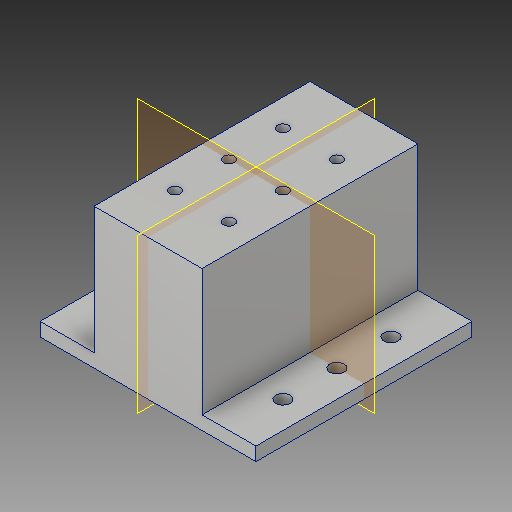
# Autodesk Inventor part: SupportPlateMotorMountV01
Saved by Autodesk Inventor 2017 (Build 210142000, 142)
## iProperties
Created: 2016-02-07
Part Number: SupportPlateMotorMountV01
Material: Aluminum 6061
Document SubType Name: Modeling
Designer: steele
Density: 2.7 g/cm^3
Appearance: Aluminum - Flat
Author: steele
Autodesk Inventor part; units mm, degrees
ref_plane "XZ Plane" through (0, 0, 0) normal (0, 1, 0) x (-1, 0, 0)
sketch "Sketch1" plane through (0, 0, 0) normal (0, 1, 0) x (-1, 0, 0)
  line L0 (50.8, 50.8) -> (-50.8, 50.8)
  line L1 (-50.8, 50.8) -> (-50.8, -50.8)
  line L2 (-50.8, -50.8) -> (50.8, -50.8)
  line L3 (50.8, -50.8) -> (50.8, 50.8)
  line L4 (50.8, 50.8) -> (-50.8, -50.8) construction
  line L5 (-50.8, 50.8) -> (50.8, -50.8) construction
  point P0 (0, 0)
  dimension "d0" = 101.6
  dimension "d1" = 101.6
  constraints: 12 end point, 2 midpoint, 2 parallel, 1 horizontal, 1 perpendicular
  measures "d0" distance of L2.end L0.start
  measures "d1" distance of L0.start L0.end
extrude "Extrusion1" add sketch "Sketch1" along normal blind 6.35
sketch "Sketch4" plane through (0, 6.35, 0) normal (0, 1, 0) x (1, 0, 0)
  line L0 (-25.4, -50.8) -> (25.4, -50.8)
  line L1 (25.4, -50.8) -> (25.4, 50.8)
  line L2 (25.4, 50.8) -> (-25.4, 50.8)
  line L3 (-25.4, 50.8) -> (-25.4, -50.8)
  line L4 (-25.4, -50.8) -> (25.4, 50.8) construction
  line L5 (25.4, -50.8) -> (-25.4, 50.8) construction
  line L6 (-50.8, 50.8) -> (-50.8, -50.8) projected
  line L7 (-50.8, -50.8) -> (50.8, -50.8) projected
  point P0 (0, 0)
  point P1 (0, 0)
  dimension "d15" = 50.8
  dimension "d16" = 25.4
  dimension "d17" = 101.6
  constraints: 12 end point, 2 midpoint, 2 parallel, 1 collinear, 1 horizontal, 1 perpendicular
  measures "d15" distance of L1.end L2.end
  measures "d16" distance between parallel lines of L3 L6
  measures "d17" distance of L2.end L0.start
extrude "Extrusion4" add sketch "Sketch4" along normal blind 59.6392
sketch "Sketch12" plane through (0, 65.9892, 0) normal (0, 1, 0) x (1, 0, 0)
  circle A0 centre (-12.7, -25.4) radius 2.5797
  line L0 (-25.4, -50.8) -> (25.4, -50.8) projected
  line L1 (-25.4, 50.8) -> (-25.4, -50.8) projected
  line L2 (-12.7, -25.4) -> (-12.7, 50.8) construction
  line L3 (-12.7, -25.4) -> (25.4, -25.4) construction
  circle A1 centre (-12.7, 0) radius 2.5797
  circle A2 centre (-12.7, 25.4) radius 2.5797
  circle A3 centre (12.7, -25.4) radius 2.5797
  circle A4 centre (12.7, 0) radius 2.5797
  circle A5 centre (12.7, 25.4) radius 2.5797
  point P0 (0, 0)
  dimension "d52" = 5.1594
  dimension "d53" = 25.4
  dimension "d54" = 12.7
  dimension "d57" = 25.4
  dimension "d60" = 25.4
  constraints: 6 centre point, 4 end point, 2 horizontal, 2 vertical, 10 other
  measures "d52" diameter of A0
  measures "d53" distance from line of L2.start L0
  measures "d54" distance from line of L2.start L1
  measures "d57" distance of L2.start A1.centre
  measures "d60" distance of L2.start A3.centre
extrude "Extrusion8" cut sketch "Sketch12" against normal through all
sketch "Sketch13" plane through (0, 6.35, 0) normal (0, 1, 0) x (1, 0, 0)
  circle A0 centre (-38.1, -25.4) radius 3.3782
  line L0 (-50.8, -50.8) -> (-25.4, -50.8) projected
  line L1 (-50.8, 50.8) -> (-50.8, -50.8) projected
  line L2 (-38.1, -25.4) -> (-38.1, 50.8) construction
  line L3 (-25.4, 50.8) -> (-50.8, 50.8) projected
  line L4 (-38.1, -25.4) -> (50.8, -25.4) construction
  line L5 (50.8, -50.8) -> (50.8, 50.8) projected
  line L6 (-38.1, 0) -> (50.8, 0) construction
  circle A1 centre (-38.1, 0) radius 3.3782
  line L7 (-38.1, 0) -> (-38.1, 76.2) construction
  line L8 (-38.1, 25.4) -> (50.8, 25.4) construction
  circle A2 centre (-38.1, 25.4) radius 3.3782
  line L9 (-38.1, 25.4) -> (-38.1, 101.6) construction
  line L10 (38.1, -25.4) -> (127, -25.4) construction
  circle A3 centre (38.1, -25.4) radius 3.3782
  line L11 (38.1, -25.4) -> (38.1, 50.8) construction
  line L12 (38.1, 0) -> (127, 0) construction
  circle A4 centre (38.1, 0) radius 3.3782
  line L13 (38.1, 0) -> (38.1, 76.2) construction
  line L14 (38.1, 25.4) -> (127, 25.4) construction
  circle A5 centre (38.1, 25.4) radius 3.3782
  line L15 (38.1, 25.4) -> (38.1, 101.6) construction
  point P0 (0, 0)
  dimension "d65" = 6.7564
  dimension "d66" = 25.4
  dimension "d67" = 12.7
  dimension "d70" = 25.4
  dimension "d73" = 76.2
  constraints: 24 end point, 6 centre point, 2 collinear, 1 horizontal, 1 midpoint, 1 perpendicular, 1 point on line, 1 vertical, 28 other
  measures "d65" diameter of A0
  measures "d66" distance from line of L2.start L0
  measures "d67" distance from line of L2.start L1
  measures "d70" distance of L2.start L6.start
  measures "d73" distance of L2.start L10.start
extrude "Extrusion9" cut sketch "Sketch13" against normal through all
equation "\"d0\" = width"
equation "\"d1\" = length"
equation "\"d2\" = thickness"
equation "\"width\" = 101.6"
equation "\"length\" = 101.6"
equation "\"thickness\" = 6.35"
body "Solid1"
